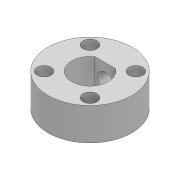
# Autodesk Inventor part: omniWheelInsert
Saved by Autodesk Inventor 2020 (Build 240168000, 168)
## iProperties
Created: 2018-06-10
Part Number: omniWheelInsert
Material: Generic
Document SubType Name: Modeling
Designer: ishaa
Density: 1 g/cm^3
Appearance: Default
Author: ishaa
Autodesk Inventor part; units mm, degrees
ref_plane "YZ Plane" through (0, 0, 0) normal (1, 0, 0) x (0, 1, 0)
ref_plane "XZ Plane" through (0, 0, 0) normal (0, 1, 0) x (-1, 0, 0)
ref_plane "XY Plane" through (0, 0, 0) normal (0, 0, 1) x (1, 0, 0)
sketch "Sketch6" plane through (0, 0, 0) normal (0, 0, 1) x (1, 0, 0)
  circle A0 centre (0, 0) radius 7.75
  dimension "d44" = 15.5
  constraints: 1 centre point, 1 coincident
  measures "d44" diameter of A0
extrude "Extrusion5" add sketch "Sketch6" along normal blind 6
sketch "Sketch7" plane through (0, 0, 0) normal (0, 0, -1) x (-1, 0, 0)
  point P0 (0, 0)
  point P1 (4.2426, 4.2426)
  point P2 (-4.2426, 4.2426)
  point P3 (-4.2426, -4.2426)
  point P4 (4.2426, -4.2426)
  dimension "d47" = 6
  dimension "d50" = 360
  dimension "d74" = 4.2426
  constraints: 5 other
  measures "d47" distance of point (4.243, 4.243) point (0, 0)
  measures "d74" horizontal distance of point (0, 0) point (4.243, 4.243)
hole "Hole4" at (-4.2426, 4.2426, 0) at (4.2426, 4.2426, 0) at (4.2426, -4.2426, 0) at (-4.2426, -4.2426, 0) direction (0, 0, 1) diameter 2.6 end through all
hole "Hole5" at (0, 0, 0) direction (0, 0, 1) diameter 6.731 end through all
sketch "Sketch8" plane through (0, 0, 0) normal (0, 0, -1) x (-1, 0, 0)
  circle A0 centre (0, 0) radius 3.3655 projected
  line L0 (-1.8762, 2.794) -> (1.8762, 2.794)
  line L1 (1.8762, 2.794) -> (1.8762, 3.429)
  line L2 (1.8762, 3.429) -> (-1.8762, 3.429)
  line L3 (-1.8762, 3.429) -> (-1.8762, 2.794)
  dimension "d70" = 2.794
  dimension "d71" = 0.635
  constraints: 8 end point, 2 parallel, 2 point on circle, 1 horizontal, 1 perpendicular
  measures "d70" distance from line of point (0, 0) L0
  measures "d71" distance between parallel lines of L0 L2
extrude "Extrusion6" add sketch "Sketch8" against normal blind 6 contours L0 A0 picked at (-0.1324, 2.9767)
sketch "Sketch9" plane through (-1.8762, 2.794, 0) normal (0, -1, 0) x (1, 0, 0)
  line L0 (0, 0) -> (0, 6) projected
  line L1 (3.7524, 0) -> (0, 0) projected
  point P0 (2, 3)
  dimension "d75" = 2
  dimension "d85" = 3
  measures "d75" distance from line of L0 point (2, 3)
  measures "d85" distance from line of L1 point (2, 3)
hole "Hole6" at (0.1238, 2.794, 3) direction (0, 1, 0) diameter 3 end through all
body "Solid2"
